Autodesk Fusion 360 part; units mm, degrees
(part 2 of 2)
  line L990 (227.5, -102.4797) -> (227.5, -114.0267)
  line L991 (227.5, -114.0267) -> (237.5, -119.8002)
  line L992 (-88, 88) -> (88, 88)
  line L993 (88, 88) -> (88, -88)
  line L994 (88, -88) -> (-88, -88)
  line L995 (-88, -88) -> (-88, 88)
  line L996 (100, 100) -> (-100, 100)
  line L997 (-100, 100) -> (-100, -100)
  line L998 (-100, -100) -> (100, -100)
  line L999 (100, -100) -> (100, 100)
  dimension "d38" = 25
  dimension "d39" = 25
  constraint coincident L6.start L7.start
  constraint midpoint L5 L6.end
  constraint midpoint L4 L7.end
extrude "Extrude6" add sketch "Sketch6" along normal up to surface (3 mm away) contours L134 L135 L138 L139 L140 L141 L144 L145 L146 L147 L150 L151 L152 L153 L156 L157 L158 L159 L162 L163 L164 L165 L168 L169 L170 L171 L174 L175 L218 L219 L220 L221 L223 L260 L262 L263 L264 L265 L392 L393 L394 L395 L397 L434 L436 L437 L438 L439 L560 L561 L562 L563 L565 L602 L604 L605 L606 L607 L734 L735 L736 L737 L739 L776 L778 L779 L780 L781 L825 L826 L827 L828 L831 L832 L833 L834 L837 L838 L839 L840 L843 L844 L845 L846 L849 L850 L851 L852 L855 L856 L857 L858 L861 L862 L863 L864 L992 L993 L994 L995 bodies 1 2
extrude "Extrude7" cut sketch "Sketch4" along normal up to surface (3 mm away) contours L6 L7 L8 L9 | L20 L21 L22 L23 | L24 L25 L26 L27 bodies 1
extrude "Extrude8" add sketch "Sketch4" along normal blind 30 contours L6 L7 L8 L9 bodies 1
fillet "Fillet2" radius 10 4 edges at (-20, 0, 3) (0, -20, 3) (20, 0, 3) (0, 20, 3) on bodies 1
extrude "Extrude9" add sketch "Sketch4" along normal up to surface (3 mm away) contours L12 L13 L17 L18 L28 L29 bodies 1
extrude "Extrude10" add sketch "Sketch4" along normal blind 3 contours L20 L21 L22 L23 bodies 1
pattern_circular "C-Pattern1" count 4 over 360 about axis through (0, 0, 1.75) along (0, 0, 1) of "Extrude9"
